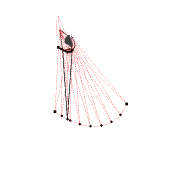
# Autodesk Inventor part: COXA_YAW_SERVO_BASE
Saved by Autodesk Inventor 2019.4 (Build 234330000, 330)
## iProperties
Created: 2019-10-21
Part Number: COXA_YAW_SERVO_BASE
Material: 一般
Document SubType Name: Modeling
Designer: y6tada
Density: 1 g/cm^3
Appearance: Black 80
Author: y6tada
Autodesk Inventor part; units mm, degrees
ref_plane "YZ Plane" through (0, 0, 0) normal (1, 0, 0) x (0, 1, 0)
ref_plane "XZ Plane" through (0, 0, 0) normal (0, 1, 0) x (-1, 0, 0)
ref_plane "XY Plane" through (0, 0, 0) normal (0, 0, 1) x (1, 0, 0)
sketch "スケッチ1" plane through (0, 0, 0) normal (0, 0, 1) x (1, 0, 0)
  line L0 (51.397, 0) -> (6, 70) construction
  line L1 (51.397, 0) -> (65, -20.9752)
  line L2 (65, -20.9752) -> (25, -44.6993)
  line L3 (0, 0) -> (0, 56.1205) construction
  line L4 (0, 0) -> (51.397, 0) construction
  arc A0 (17.9848, 26.067) -> (17.1698, 21.0636) centre (51.7641, 17.9963) ccw construction
  arc A1 (10.2038, 27.926) -> (9.201, 21.7701) centre (51.7641, 17.9963) ccw construction
  arc A2 (9.201, 21.7701) -> (17.1698, 21.0636) centre (13.1854, 21.4169) ccw construction
  line L5 (13.1854, 21.4169) -> (51.7641, 17.9963) construction
  line L6 (51.7641, 17.9963) -> (13.5604, 24.3596)
  arc A3 (13.5604, 24.3596) -> (13.1854, 21.4169) centre (51.7641, 17.9963) ccw construction
  line L7 (13.1854, 21.4169) -> (66.7927, -23.5971) construction
  line L8 (66.7927, -23.5971) -> (61.9625, 22.6577) construction
  line L9 (13.5604, 24.3596) -> (25, -44.6993)
  line L10 (13.5604, 24.3596) -> (6, 70) construction
  line L11 (13.5604, 24.3596) -> (51.397, 0) construction
  arc A4 (51.397, -25) -> (61.9625, 22.6577) centre (51.397, 0) ccw
  line L12 (25, -44.6993) -> (65, -44.6993) construction
  line L13 (65, -44.6993) -> (65, -20.9752) construction
  line L14 (45, -44.6993) -> (45, -284.6993) construction
  line L15 (51.397, 0) -> (51.9579, -2.4363)
  line L16 (51.397, 0) -> (50.5419, -2.3492) construction
  arc A5 (50.5419, -2.3492) -> (53.1648, 1.7678) centre (51.397, 0) ccw construction
  line L17 (51.397, 0) -> (51.3697, -2.4999) construction
  line L18 (51.397, 0) -> (52.2006, -2.3673) construction
  line L19 (51.397, 0) -> (52.9404, -1.9667) construction
  line L20 (51.397, 0) -> (53.5055, -1.3432) construction
  line L21 (51.397, 0) -> (53.8317, -0.5677) construction
  line L22 (51.397, 0) -> (53.8821, 0.2722) construction
  line L23 (51.397, 0) -> (53.6511, 1.0812) construction
  line L24 (51.397, 0) -> (53.1648, 1.7678) construction
  line L25 (51.7641, 17.9963) -> (51.9579, -2.4363)
  line L26 (50.5419, -2.3492) -> (51.7641, 17.9963) construction
  line L27 (51.7641, 17.9963) -> (53.1648, 1.7678) construction
  line L28 (51.397, -8) -> (51.397, -25) construction
  line L29 (54.051, -7.5469) -> (59.6907, -23.5842) construction
  line L30 (56.4044, -6.2391) -> (67.0451, -19.4971) construction
  line L31 (58.1906, -4.2245) -> (72.6271, -13.2017) construction
  line L32 (59.2074, -1.7315) -> (75.8044, -5.411) construction
  line L33 (59.3395, 0.9576) -> (76.2172, 2.9926) construction
  line L34 (58.572, 3.5383) -> (73.8188, 11.0572) construction
  line L35 (56.9918, 5.7182) -> (68.8808, 17.8694) construction
  line L36 (54.7779, 7.2505) -> (61.9625, 22.6577) construction
  arc A6 (51.397, -8) -> (54.7779, 7.2505) centre (51.397, 0) ccw construction
  line L37 (14.0943, 26.9965) -> (51.7641, 17.9963) construction
  arc A7 (14.0943, 26.9965) -> (13.5604, 24.3596) centre (51.7641, 17.9963) ccw construction
  arc A8 (17.9848, 26.067) -> (10.2038, 27.926) centre (14.0943, 26.9965) ccw construction
  line L38 (51.3697, -2.4999) -> (51.7641, 17.9963) construction
  line L39 (51.7641, 17.9963) -> (13.7589, 25.4541) construction
  line L40 (13.4871, 23.9026) -> (51.7641, 17.9963) construction
  line L41 (52.2006, -2.3673) -> (51.7641, 17.9963) construction
  line L42 (14.0943, 26.9965) -> (8.4208, -42.7732) construction
  line L43 (8.4208, -42.7732) -> (51.397, -25) construction
  line L44 (13.7589, 25.4541) -> (18.1084, -44.4107) construction
  line L45 (18.1084, -44.4107) -> (59.6907, -23.5842) construction
  line L46 (25, -44.6993) -> (45, -284.6993)
  line L47 (65, -20.9752) -> (45, -284.6993)
  line L48 (18.1084, -44.4107) -> (21.0305, -285.2248) construction
  line L49 (21.0305, -285.2248) -> (59.6907, -23.5842) construction
  line L50 (51.397, -25) -> (-6.0328, -283.171) construction
  line L51 (-6.0328, -283.171) -> (8.4208, -42.7732) construction
  line L52 (51.7641, 17.9963) -> (13.2929, 22.4663) construction
  line L53 (51.7641, 17.9963) -> (13.173, 21.2739) construction
  line L54 (51.7641, 17.9963) -> (13.1124, 20.4583) construction
  line L55 (51.7641, 17.9963) -> (13.0939, 20.1483) construction
  line L56 (51.7641, 17.9963) -> (13.1119, 20.4513) construction
  line L57 (51.7641, 17.9963) -> (52.9404, -1.9667) construction
  line L58 (51.7641, 17.9963) -> (53.5055, -1.3432) construction
  line L59 (51.7641, 17.9963) -> (53.8317, -0.5677) construction
  line L60 (51.7641, 17.9963) -> (53.8821, 0.2722) construction
  line L61 (51.7641, 17.9963) -> (53.6511, 1.0812) construction
  line L62 (13.4871, 23.9026) -> (27.8947, -44.5986) construction
  line L63 (27.8947, -44.5986) -> (67.0451, -19.4971) construction
  line L64 (72.6271, -13.2017) -> (37.1961, -43.3261) construction
  line L65 (37.1961, -43.3261) -> (13.2929, 22.4663) construction
  line L66 (13.173, 21.2739) -> (45.5916, -40.7666) construction
  line L67 (45.5916, -40.7666) -> (75.8044, -5.411) construction
  line L68 (76.2172, 2.9926) -> (52.8124, -37.1951) construction
  line L69 (52.8124, -37.1951) -> (13.1124, 20.4583) construction
  line L70 (13.0939, 20.1483) -> (58.7276, -32.9324) construction
  line L71 (58.7276, -32.9324) -> (73.8188, 11.0572) construction
  line L72 (68.8808, 17.8694) -> (63.3391, -28.3055) construction
  line L73 (63.3391, -28.3055) -> (13.1119, 20.4513) construction
  line L74 (27.8947, -44.5986) -> (56.2327, -283.7575) construction
  line L75 (61.9625, 22.6577) -> (293.1766, -105.7574) construction
  line L76 (293.1766, -105.7574) -> (66.7927, -23.5971) construction
  line L77 (68.8808, 17.8694) -> (265.8829, -158.5975) construction
  line L78 (265.8829, -158.5975) -> (63.3391, -28.3055) construction
  line L79 (58.7276, -32.9324) -> (229.4847, -202.7618) construction
  line L80 (229.4847, -202.7618) -> (73.8188, 11.0572) construction
  line L81 (76.2172, 2.9926) -> (187.0489, -237.1465) construction
  line L82 (187.0489, -237.1465) -> (52.8124, -37.1951) construction
  line L83 (45.5916, -40.7666) -> (141.9163, -261.4962) construction
  line L84 (141.9163, -261.4962) -> (75.8044, -5.411) construction
  line L85 (72.6271, -13.2017) -> (97.3466, -276.5254) construction
  line L86 (97.3466, -276.5254) -> (37.1961, -43.3261) construction
  line L87 (56.2327, -283.7575) -> (67.0451, -19.4971) construction
  spline S0 degree 4 poles (-6.0328, -283.171) (-1.0018, -286.6814) (51.7016, -283.757) (37.9506, -286.9352) (110.0397, -275.596) (142.8766, -261.8211) (210.6869, -227.817) (251.1, -183.7947) (281.212, -139.9837) (293.1766, -105.7574) knots 0 0 0 0 0 0.215081 0.31035 0.415619 0.538699 0.666654 1 1 1 1 1 construction
  spline S1 degree 4 poles (8.4208, -42.7732) (14.2837, -44.205) (22.8164, -45.2788) (33.6178, -44.6875) (45.3572, -41.166) (55.0356, -36.4401) (61.2363, -31.2275) (64.7888, -26.7723) (66.7927, -23.5971) knots 0 0 0 0 0 0.340062 0.471566 0.598373 0.71961 1 1 1 1 1
  point P0 (51.397, 0)
  point P1 (51.397, 0)
  point P2 (51.397, 0)
  point P3 (51.397, 0)
  point P4 (51.397, 0)
  point P5 (51.397, 0)
  point P6 (51.397, 0)
  point P7 (51.397, 0)
  dimension "d5" = 70
  dimension "d53" = 45
  dimension "d66" = 25
  dimension "d67" = 40
  dimension "d72" = 240
  dimension "d74" = 20
  dimension "d76" = 2.5
  dimension "d80" = 155
  dimension "d82" = 18
  dimension "d85" = 155
  dimension "d87" = 20
  dimension "d88" = 70
  dimension "d89" = 100
  dimension "d90" = 100
  dimension "d91" = 100
  dimension "d92" = 4
  dimension "d93" = 100
  dimension "d94" = 100
  dimension "d95" = 90
  dimension "d96" = 100
  dimension "d97" = 100
  dimension "d98" = 100
  dimension "d99" = 100
  dimension "d100" = 100
  dimension "d101" = 8
  dimension "d102" = 6
  dimension "d103" = 45
  constraints: 176 end point, 36 equal length, 28 point on circle, 16 coincident, 14 point on line, 9 centre point, 4 tangent, 2 horizontal, 2 midpoint, 2 vertical, 1 collinear, 1 concentric, 1 perpendicular, 76 other
  measures "d5" distance from line of L4 L0.end
  measures "d53" distance of L6.end L11.end
  measures "d66" radius of A4
  measures "d67" distance of L2.end L12.end
  measures "d72" distance of L14.start L14.end
  measures "d74" angle of L15 L1
  measures "d76" radius of A5
  measures "d82" distance of L0.start L5.end
  measures "d87" angle of L16 L28
  measures "d88" distance of L6.end L2.end
  measures "d89" angle of L25 L6
  measures "d90" angle of L26 L37
  measures "d91" angle of L27 L5
  measures "d92" radius of A8
  measures "d93" angle of L38 L39
  measures "d94" angle of L40 L41
  measures "d95" angle of L28 L4
  measures "d96" angle of L57 L52
  measures "d97" angle of L58 L53
  measures "d98" angle of L59 L54
  measures "d99" angle of L55 L60
  measures "d100" angle of L61 L56
  measures "d101" radius of A6
  measures "d102" distance from line of L0.end L3
  measures "d103" distance between parallel lines of L14 L3
sketch "スケッチ2" plane through (0, 0, 0) normal (0, 0, 1) x (1, 0, 0)
  arc A0 (55.0538, 20.2717) -> (48.4917, 20.2966) centre (51.7641, 17.9963) ccw
  line L0 (40, 3) -> (64, 3) construction
  line L1 (64, 3) -> (64, -9) construction
  line L2 (64, -9) -> (40, -9) construction
  line L3 (40, -9) -> (40, 3) construction
  line L4 (36, 10.1673) -> (36, -48.9437) construction
  line L5 (67, 3) -> (67, -9)
  line L6 (64, -12) -> (40, -12)
  line L7 (37, -9) -> (37, 3)
  arc A1 (37, -9) -> (40, -12) centre (40, -9) ccw
  arc A2 (37.5457, 4.7253) -> (37, 3) centre (40, 3) ccw
  arc A3 (64, -12) -> (67, -9) centre (64, -9) ccw
  line L8 (0, 0) -> (0, -59.5537) construction
  line L9 (10.6628, -3) -> (66.9205, -3) construction
  line L10 (67, 3) -> (55.0538, 20.2717)
  line L11 (37.5457, 4.7253) -> (48.4917, 20.2966)
  dimension "d16" = 24
  dimension "d17" = 4
  dimension "d18" = 12
  dimension "d19" = 3
  dimension "d20" = 72
  dimension "d21" = 3
  dimension "d23" = 4
  constraints: 24 end point, 8 point on circle, 8 tangent, 4 centre point, 3 coincident, 3 horizontal, 3 parallel, 3 vertical, 2 equal radius, 1 perpendicular, 1 other
  measures "d16" distance of L1.end L2.end
  measures "d17" distance between parallel lines of L3 L4
  measures "d18" distance of L2.end L0.start
  measures "d19" radius of A1
  measures "d20" diameter of L4 L8
  measures "d21" distance from line of L8.start L9
  measures "d23" radius of A0
extrude "押し出し1" add sketch "スケッチ2" along normal blind 2
hole "穴1" at (51.7641, 17.9963, 0) direction (0, 0, 1) diameter 3 end through all
hole "穴2" at (64, 3, 0) at (40, 3, 0) at (40, -9, 0) at (64, -9, 0) direction (0, 0, 1) diameter 2.5 end through all
equation "\"input_link_length\" = 25"
equation "\"input_link_formed_angle\" = 20deg"
equation "\"support_formed_angle\" = 100deg"
equation "\"input_slider_radius\" = 2.5"
equation "\"driver_rotation_range\" = 155deg"
equation "\"virtual_link_length\" = 45"
equation "\"virtual_mass_point_x\" = 6"
equation "\"support_axis_driver_dist\" = 18"
